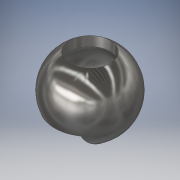
# Autodesk Inventor part: Шар Модель Ауд
Saved by Autodesk Inventor 2019 (Build 230136000, 136)
## iProperties
Created: 2020-04-11
Part Number: Шар Модель Ауд
Material: Сталь, высокопрочная, низколегированная
Document SubType Name: Modeling
Designer: Ivan
Mass: 178.335 g
Surface Area: 104.585 cm^2
Volume: 22.7179 cm^3
Density: 7.85 g/cm^3
Appearance: Сталь — полированная
Author: Ivan
Autodesk Inventor part; units mm, degrees
ref_plane "YZ Plane" through (0, 0, 0) normal (1, 0, 0) x (0, 1, 0)
ref_plane "XZ Plane" through (0, 0, 0) normal (0, 1, 0) x (-1, 0, 0)
ref_plane "XY Plane" through (0, 0, 0) normal (0, 0, 1) x (1, 0, 0)
sketch "Эскиз1" plane through (0, 0, 0) normal (0, 0, 1) x (1, 0, 0)
  arc A0 (25, 0) -> (-25, 0) centre (0, 0) ccw
  arc A1 (20, 0) -> (-20, 0) centre (0, 0) ccw
  line L0 (-35, 0) -> (35, 0) projected
  dimension "d0" = 50
  dimension "d1" = 40
  constraints: 4 point on circle, 4 point on line, 2 centre point, 2 coincident
  measures "d0" diameter of A0
  measures "d1" diameter of A1
revolve "Вращение1" add sketch "Эскиз1" angle 360 about axis through (-10, 0, 0) along (1, 0, 0) contours L0 A1 A0
sketch "Эскиз2" plane through (0, 0, 0) normal (0, 0, 1) x (1, 0, 0)
  line L0 (-13, -10) -> (13, -10)
  line L1 (13, -10) -> (13, -25)
  line L2 (13, -25) -> (-13, -25)
  line L3 (-13, -25) -> (-13, -10)
  circle A0 centre (0, 0) radius 25 projected
  dimension "d4" = 10
  dimension "d5" = 26
  dimension "d6" = 13
  constraints: 8 end point, 2 parallel, 1 horizontal, 1 perpendicular, 1 tangent
  measures "d4" distance from line of point (0, 0) L0
  measures "d5" distance between parallel lines of L1 L3
  measures "d6" distance from line of point (0, 0) L3
extrude "Выдавливание1" cut sketch "Эскиз2" along normal through all both and the other way through all contours L0 L1 A0 L3 | A0 L2 L3 | L1 L2 A0 picked at (0, -15)
sketch "Эскиз3" plane through (0, 0, 0) normal (0, 1, 0) x (-1, 0, 0)
  circle A0 centre (0, 0) radius 13
  dimension "d9" = 26
  constraints: 1 centre point, 1 coincident
  measures "d9" diameter of A0
extrude "Выдавливание2" cut sketch "Эскиз3" along normal through all
equation "\"d6\" = 0.5 * d5"
